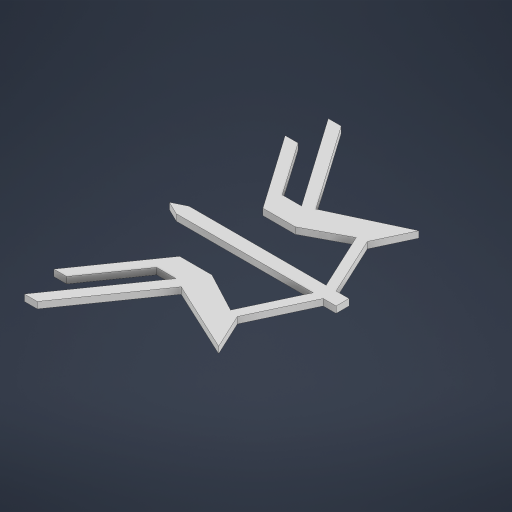
# Autodesk Inventor part: QQI
Saved by Autodesk Inventor 2024.3 (Build 283343000, 343)
## iProperties
Created: 2025-08-01
Part Number: QQI
Material: Generic
Document SubType Name: Modeling
Designer: LeoFB
Density: 1 g/cm^3
Appearance: Default
Author: LeoFB
Autodesk Inventor part; units mm, degrees
ref_plane "YZ Plane" through (0, 0, 0) normal (1, 0, 0) x (0, 1, 0)
ref_plane "XZ Plane" through (0, 0, 0) normal (0, 1, 0) x (-1, 0, 0)
ref_plane "XY Plane" through (0, 0, 0) normal (0, 0, 1) x (1, 0, 0)
sketch "Sketch1" plane through (0, 0, 0) normal (0, 1, 0) x (-1, 0, 0)
  line L0 (0, 0) -> (10, 0) construction
  line L1 (-10, 0) -> (-10, 5)
  line L2 (-10, 5) -> (0, 5)
  line L3 (-10, 0) -> (-10, -5)
  line L4 (-10, 0) -> (-5, 0) construction
  line L5 (-10, -5) -> (0, -5)
  line L6 (0, -5) -> (21.1309, -50.3154)
  line L7 (21.1309, -50.3154) -> (8.4524, -77.5046)
  line L8 (8.4524, -77.5046) -> (62.8308, -52.1475)
  line L9 (62.8308, -52.1475) -> (108.7169, -117.6797)
  line L10 (108.7169, -117.6797) -> (118.7169, -117.6797)
  line L11 (118.7169, -117.6797) -> (70.3694, -48.6322)
  line L12 (70.3694, -48.6322) -> (85.3694, -48.6322)
  line L13 (85.3694, -48.6322) -> (114.0482, -89.5898)
  line L14 (114.0482, -89.5898) -> (124.0482, -89.5898)
  line L15 (124.0482, -89.5898) -> (83.8979, -32.2492)
  line L16 (83.8979, -32.2492) -> (58.8979, -32.2492)
  line L17 (58.8979, -32.2492) -> (28.0903, -48.6322)
  line L18 (28.0903, -48.6322) -> (7.7442, -5)
  line L19 (7.7442, -5) -> (113.7169, -5)
  line L20 (113.7169, -5) -> (124.0482, 0)
  line L21 (-10, 0) -> (-10, 5)
  line L22 (-10, 5) -> (0, 5)
  line L23 (0, 5) -> (21.1309, 50.3154)
  line L24 (21.1309, 50.3154) -> (8.4524, 77.5046)
  line L25 (8.4524, 77.5046) -> (62.8308, 52.1475)
  line L26 (62.8308, 52.1475) -> (108.7169, 117.6797)
  line L27 (108.7169, 117.6797) -> (118.7169, 117.6797)
  line L28 (118.7169, 117.6797) -> (70.3694, 48.6322)
  line L29 (70.3694, 48.6322) -> (85.3694, 48.6322)
  line L30 (85.3694, 48.6322) -> (114.0482, 89.5898)
  line L31 (114.0482, 89.5898) -> (124.0482, 89.5898)
  line L32 (124.0482, 89.5898) -> (83.8979, 32.2492)
  line L33 (83.8979, 32.2492) -> (58.8979, 32.2492)
  line L34 (58.8979, 32.2492) -> (28.0903, 48.6322)
  line L35 (28.0903, 48.6322) -> (7.7442, 5)
  line L36 (7.7442, 5) -> (113.7169, 5)
  line L37 (113.7169, 5) -> (124.0482, 0)
  dimension "d2" = 5
  dimension "d4" = 10
  dimension "d6" = 5
  dimension "d7" = 90
  dimension "d8" = 10
  dimension "d9" = 90
  dimension "d10" = 50
  dimension "d12" = 30
  dimension "d13" = 130
  dimension "d14" = 60
  dimension "d15" = 80
  dimension "d16" = 100
  dimension "d17" = 10
  dimension "d18" = 125
  dimension "d19" = 15
  dimension "d20" = 55
  dimension "d21" = 50
  dimension "d22" = 125
  dimension "d23" = 10
  dimension "d24" = 125
  dimension "d25" = 70
  dimension "d26" = 55
  constraints: 76 end point, 6 parallel, 6 point on line, 4 horizontal, 4 perpendicular, 1 vertical
  measures "d2" distance of L1.start L1.end
  measures "d4" distance of L1.end L2.end
  measures "d6" distance of L1.start L3.end
  measures "d7" angle of L3 L4
  measures "d8" distance of L3.end L5.end
  measures "d9" angle of L5 L3
  measures "d10" distance of L5.end L6.end
  measures "d12" distance of L6.end L7.end
  measures "d13" angle of L6 L7
  measures "d14" distance of L7.end L8.end
  measures "d15" distance of L8.end L9.end
  measures "d16" angle of L8 L9
  measures "d17" distance of L9.end L10.end
  measures "d18" angle of L10 L9
  measures "d19" distance of L11.end L12.end
  measures "d20" angle of L11 L12
  measures "d21" distance of L12.end L13.end
  measures "d22" angle of L12 L13
  measures "d23" distance of L13.end L14.end
  measures "d24" angle of L14 L13
  measures "d25" distance of L14.end L15.end
  measures "d26" angle of L15 L14
extrude "Extrusion1" add sketch "Sketch1" along normal blind 5
body "Solid1"
